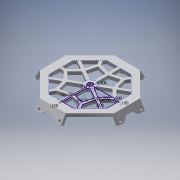
# Autodesk Inventor part: 4-Tool_Lower
Saved by Autodesk Inventor 2019 (Build 230136000, 136)
## iProperties
Created: 2021-01-31
Part Number: 4-Tool_Lower
Material: ABS Plastic
Document SubType Name: Modeling
Designer: zhanb
Density: 1.06 g/cm^3
Appearance: Smooth - White
Author: zhanb
Autodesk Inventor part; units mm, degrees
ref_plane "YZ Plane" through (0, 0, 0) normal (1, 0, 0) x (0, 1, 0)
ref_plane "XZ Plane" through (0, 0, 0) normal (0, 1, 0) x (-1, 0, 0)
ref_plane "XY Plane" through (0, 0, 0) normal (0, 0, 1) x (1, 0, 0)
sketch "Sketch1" plane through (0, 0, 0) normal (1, 0, 0) x (0, 1, 0)
  line L0 (76.2, -25.4) -> (50.8, -25.4) construction
  line L1 (50.8, -25.4) -> (50.8, 25.4) construction
  line L2 (50.8, 25.4) -> (76.2, 25.4) construction
  line L3 (76.2, 25.4) -> (76.2, -25.4) construction
  line L4 (76.2, -25.4) -> (50.8, 25.4) construction
  line L5 (50.8, -25.4) -> (76.2, 25.4) construction
  line L6 (76.2, 25.4) -> (-22.7867, 82.55) construction
  line L7 (-22.7867, 82.55) -> (-9.5885, 74.93)
  line L8 (-22.7867, 82.55) -> (-25.9617, 77.0507)
  line L9 (-25.9617, 77.0507) -> (-12.7635, 69.4307)
  line L10 (-9.5885, 74.93) -> (-12.7635, 69.4307) construction
  line L11 (-12.7635, 69.4307) -> (-12.7635, 57.15)
  line L12 (-12.7635, 57.15) -> (-6.4135, 57.15)
  line L13 (-6.4135, 57.15) -> (-6.4135, 73.0969)
  line L14 (-9.5885, 74.93) -> (-6.4135, 73.0969)
  point P0 (0, 0)
  point P1 (63.5, 0)
  point P2 (-16.1876, 78.74)
  dimension "d0" = 50.8
  dimension "d1" = 25.4
  dimension "d2" = 63.5
  dimension "d3" = 30
  dimension "d4" = 114.3
  dimension "d5" = 15.24
  dimension "d6" = 106.68
  dimension "d7" = 6.35
  dimension "d14" = 6.35
  dimension "d65" = 57.15
  constraints: 30 end point, 6 perpendicular, 3 midpoint, 2 parallel, 2 point on line, 1 collinear, 1 horizontal, 1 horizontal alignment, 1 vertical
  measures "d0" distance of L2.end L0.start
  measures "d1" distance of L1.end L2.end
  measures "d2" distance of point (0, 0) point (63.5, 0)
  measures "d3" angle of L2 L6
  measures "d4" distance of L2.end L6.end
  measures "d5" distance of L6.end L7.end
  measures "d6" distance of L2.end point (-16.188, 78.74)
  measures "d7" distance between parallel lines of L6 L9
  measures "d14" distance of L11.end L12.end
  measures "d65" distance from line of L12 point (0, 0)
extrude "Extrusion1" add sketch "Sketch1" along normal mid plane 50.8
pattern_circular "Circular Pattern1" count 4 over 360 about axis through (0, -10, 0) along (0, 1, 0) of "Extrusion1"
sketch "Sketch2" plane through (-25.4, -6.4135, 73.0969) normal (0, 1, 0) x (1, 0, 0)
  line L0 (50.8, 0) -> (0, 0) construction
  line L1 (50.8, 15.9469) -> (50.8, 0) construction
  line L2 (50.8, 15.9469) -> (0, 15.9469) construction
  line L3 (0, 0) -> (0, 15.9469) construction
  line L4 (-47.6969, 47.6969) -> (-47.6969, 98.4969) construction
  line L5 (-31.75, 47.6969) -> (-47.6969, 47.6969) construction
  line L6 (-31.75, 47.6969) -> (-31.75, 98.4969) construction
  line L7 (-47.6969, 98.4969) -> (-31.75, 98.4969) construction
  line L8 (-47.6969, 47.6969) -> (0, 0)
  line L9 (-44.0307, 47.6969) -> (-31.75, 47.6969) projected
  line L10 (-47.6969, 47.6969) -> (-31.75, 47.6969)
  line L11 (0, 0) -> (0, 15.9469)
  line L12 (0, 3.6662) -> (0, -3.9538) projected
  line L13 (0, 15.9469) -> (1.7277, 15.9469)
  line L14 (50.8, 15.9469) -> (0, 15.9469) projected
  line L15 (1.7277, 15.9469) -> (-31.75, 49.4246)
  line L16 (-31.75, 47.6969) -> (-31.75, 98.4969) projected
  line L17 (-31.75, 49.4246) -> (-31.75, 47.6969)
  point P0 (25.4, 73.0969)
  dimension "d64" = 57.15
  constraints: 12 end point, 2 collinear, 2 point on line, 1 horizontal, 1 parallel
  measures "d64" distance from line of L15 point (25.4, 73.097)
extrude "Extrusion2" add sketch "Sketch2" against normal up to surface (6.35 mm away)
sketch "Sketch3" plane through (-25.4, -22.7867, 82.55) normal (0, 0.5, 0.8660254) x (1, 0, 0)
  line L0 (50.8, 0) -> (0, 0) construction
  line L1 (10.16, 0) -> (18.034, 7.874)
  line L2 (18.034, 7.874) -> (32.766, 7.874)
  line L3 (32.766, 7.874) -> (40.64, 0)
  line L4 (10.16, 0) -> (40.64, 0)
  line L5 (5.08, 5.08) -> (45.72, 5.08) construction
  line L6 (0, 0) -> (0, 18.9062) construction
  line L7 (50.8, 18.9062) -> (50.8, 0) construction
  point P0 (25.4, 61.0089)
  point P1 (25.4, 7.874)
  point P2 (25.4, 0)
  dimension "d19" = 45
  dimension "d20" = 10.16
  dimension "d21" = 7.874
  dimension "d24" = 5.08
  dimension "d25" = 5.08
  dimension "d26" = 5.08
  constraints: 10 end point, 2 midpoint, 2 parallel, 2 point on line, 1 horizontal, 1 perpendicular, 1 vertical alignment
  measures "d19" angle of L0 L1
  measures "d20" distance of L0.end L1.start
  measures "d21" distance between parallel lines of L0 L2
  measures "d24" distance from line of L0 L5.start
  measures "d25" distance from line of L6 L5.start
  measures "d26" distance from line of L7 L5.end
extrude "Extrusion3" cut sketch "Sketch3" against normal through all
hole "Hole1" at (-20.32, -18.3873, 80.01) at (20.32, -18.3873, 80.01) direction (0, -0.5, -0.8660254) diameter 5.1562 end through all
sketch "Sketch5" plane through (0, 0, 0) normal (1, 0, 0) x (0, 1, 0)
  line L0 (-12.7635, 69.4307) -> (-25.9617, 77.0507) construction
  line L1 (-12.7635, 25.4) -> (-12.7635, 73.0969) projected
  line L2 (-19.1135, 73.0969) -> (-19.1135, 61.6669)
  line L3 (-19.1135, 61.6669) -> (-12.7635, 58.0007)
  line L4 (-12.7635, 69.4307) -> (-12.7635, 57.15) projected
  line L5 (-12.7635, 69.4307) -> (-19.1135, 73.0969)
  line L6 (-19.1426, 73.1137) -> (-25.9617, 77.0507) projected
  line L7 (-12.7635, 69.4307) -> (-12.7635, 58.0007)
  point P0 (0, 0)
  dimension "d34" = 6.35
  dimension "d35" = 11.43
  constraints: 8 end point, 2 collinear, 2 point on line, 1 parallel, 1 vertical
  measures "d34" distance between parallel lines of L1 L2
  measures "d35" distance of L2.start L2.end
extrude "Extrusion4" add sketch "Sketch5" along normal mid plane 5.08
pattern_circular "Circular Pattern2" count 4 over 360 about axis through (0, -10, 0) along (0, 1, 0) of "Extrusion4", "Extrusion3", "Hole1", "Extrusion2"
sketch "Sketch6" plane through (-25.4, -6.4135, 73.0969) normal (0, 1, 0) x (1, 0, 0)
  line L0 (20.6121, 70.3326) -> (20.6121, 75.8612) construction
  line L1 (20.6121, 75.8612) -> (25.4, 78.6255) construction
  line L2 (25.4, 78.6255) -> (30.1879, 75.8612) construction
  line L3 (30.1879, 75.8612) -> (30.1879, 70.3326) construction
  line L4 (30.1879, 70.3326) -> (25.4, 67.5683) construction
  line L5 (25.4, 67.5683) -> (20.6121, 70.3326) construction
  line L6 (82.55, 49.4246) -> (78.4987, 45.3733)
  line L7 (78.4987, 45.3733) -> (59.9942, 56.0569)
  line L8 (35.2679, 70.3326) -> (35.2679, 73.0969)
  line L9 (35.2679, 73.0969) -> (69.85, 73.0969)
  line L10 (82.55, 73.0969) -> (82.55, 70.5569) construction
  line L11 (32.7279, 65.9332) -> (52.8996, 54.2871)
  line L12 (74.7799, 41.6545) -> (56.8424, 23.717)
  line L13 (49.0723, 15.9469) -> (27.94, 15.9469)
  line L14 (27.94, 15.9469) -> (27.94, 34.6175)
  line L15 (27.94, 63.1689) -> (32.7279, 65.9332)
  line L16 (82.55, 96.7692) -> (82.55, 49.4246) construction
  line L17 (82.55, 49.4246) -> (53.1236, 19.9982) construction
  line L18 (49.0723, 15.9469) -> (1.7277, 15.9469) construction
  line L19 (1.7277, 15.9469) -> (-31.75, 49.4246) construction
  line L20 (-31.75, 49.4246) -> (-31.75, 96.7692) construction
  line L21 (-31.75, 96.7692) -> (1.7277, 130.2469) construction
  line L22 (1.7277, 130.2469) -> (49.0723, 130.2469) construction
  line L23 (49.0723, 130.2469) -> (82.55, 96.7692) construction
  line L24 (82.55, 96.7692) -> (82.55, 49.4246) construction
  line L25 (30.1879, 70.3326) -> (76.6393, 43.5139) construction
  line L26 (35.2679, 78.7941) -> (35.2679, 67.3997) construction
  line L27 (35.2679, 67.3997) -> (25.4, 61.7024) construction
  line L28 (25.4, 61.7024) -> (15.5321, 67.3997) construction
  line L29 (15.5321, 67.3997) -> (15.5321, 78.7941) construction
  line L30 (15.5321, 78.7941) -> (25.4, 84.4914) construction
  line L31 (25.4, 84.4914) -> (35.2679, 78.7941) construction
  line L32 (82.55, 70.5569) -> (74.4942, 70.5569)
  line L33 (74.4942, 70.5569) -> (59.9942, 56.0569)
  line L34 (55.4396, 58.6865) -> (69.85, 73.0969)
  line L35 (69.85, 73.0969) -> (82.55, 73.0969) construction
  line L36 (82.55, 70.5569) -> (82.55, 49.4246)
  line L37 (55.4396, 58.6865) -> (35.2679, 70.3326)
  line L38 (59.9942, 56.0569) -> (55.4396, 58.6865) construction
  line L39 (52.8996, 54.2871) -> (47.625, 34.6021)
  line L40 (47.625, 34.6021) -> (27.94, 39.8767)
  line L41 (57.4542, 51.6575) -> (52.1468, 31.8501)
  line L42 (52.1468, 31.8501) -> (56.8424, 23.717)
  line L43 (27.94, 34.6175) -> (47.7474, 29.3101)
  line L44 (47.7474, 29.3101) -> (53.1236, 19.9982)
  line L45 (54.983, 21.8576) -> (30.3339, 64.5511) construction
  line L46 (52.1468, 31.8501) -> (47.625, 34.6021) construction
  line L47 (47.625, 34.6021) -> (47.7474, 29.3101) construction
  line L48 (47.7474, 29.3101) -> (52.1468, 31.8501) construction
  line L49 (55.4396, 58.6865) -> (52.8996, 54.2871) construction
  line L50 (52.8996, 54.2871) -> (57.4542, 51.6575) construction
  line L51 (57.4542, 51.6575) -> (74.7799, 41.6545)
  line L52 (27.94, 39.8767) -> (27.94, 63.1689)
  line L53 (27.94, 34.6175) -> (27.94, 39.8767) construction
  line L54 (56.8424, 23.717) -> (53.1236, 19.9982) construction
  line L55 (53.1236, 19.9982) -> (49.0723, 15.9469) construction
  line L56 (53.1236, 19.9982) -> (49.0723, 15.9469)
  circle A0 centre (25.4, 73.0969) radius 4.7879
  line L57 (82.55, 49.4246) -> (49.0723, 15.9469) construction
  line L58 (27.94, 15.9469) -> (25.4, 15.9469)
  line L59 (25.4, 15.9469) -> (25.4, 61.7024)
  line L60 (25.4, 61.7024) -> (25.4, 68.309)
  line L61 (69.85, 73.0969) -> (82.55, 73.0969)
  line L62 (82.55, 73.0969) -> (82.55, 70.5569)
  line L63 (35.2679, 73.0969) -> (30.1879, 73.0969)
  arc A1 (25.4, 68.309) -> (30.1879, 73.0969) centre (25.4, 73.0969) ccw
  line L64 (53.1236, 19.9982) -> (56.8424, 23.717)
  line L65 (78.4987, 45.3733) -> (74.7799, 41.6545)
  point P0 (25.4, 73.0969)
  point P1 (27.794, 68.9505)
  point P2 (27.7939, 77.2434)
  dimension "d41" = 9.5758
  dimension "d42" = 2.54
  dimension "d43" = 5.08
  dimension "d45" = 30
  dimension "d46" = 5.08
  dimension "d48" = 5.08
  dimension "d49" = 2.54
  dimension "d50" = 5.08
  dimension "d51" = 5.08
  dimension "d52" = 5.08
  dimension "d61" = 12.7
  constraints: 128 end point, 17 parallel, 13 collinear, 13 point on line, 7 midpoint, 7 perpendicular, 5 coincident, 5 point on circle, 5 vertical, 3 horizontal, 2 centre point, 1 equal length, 46 other
  measures "d41" distance between parallel lines of L0 L3
  measures "d42" distance from line of L4.end L14
  measures "d43" distance between parallel lines of L7 L11
  measures "d45" angle of L9 L25
  measures "d46" distance between parallel lines of L26 L3
  measures "d48" distance between parallel lines of L34 L33
  measures "d49" distance between parallel lines of L35 L32
  measures "d50" distance between parallel lines of L44 L42
  measures "d51" distance between parallel lines of L39 L41
  measures "d52" distance between parallel lines of L43 L40
  measures "d61" distance of L10.start L9.end
extrude "Extrusion6" add sketch "Sketch6" against normal up to surface (6.35 mm away) contours L65 L51 L41 L42 L64 L44 L43 L14 L58 L59 L60 A0 L63 L8 L37 L34 L61 L62 L32 L33 L7
mirror "Mirror1" about plane through (0, 0, 0) normal (1, 0, 0) of "Extrusion6"
mirror "Mirror2" about plane through (0, 0, 0) normal (0, 0, 1) of "Extrusion6", "Mirror1"
fillet "Fillet2" radius 1.5875 50 edges at (-2.54, -9.5885, -33.2202) (-22.225, -9.5885, -38.4948) (-2.54, -9.5885, -9.928) (-2.54, -9.5885, -38.4795) (-22.3474, -9.5885, -43.7868) (-26.7468, -9.5885, -41.2468) (-32.0542, -9.5885, -21.4394) (-7.3279, -9.5885, -7.1637) (-27.4996, -9.5885, -18.8098) (-34.5942, -9.5885, -17.04) (-49.0942, -9.5885, -2.54) (-30.0396, -9.5885, -14.4104) (22.225, -9.5885, -38.4948) (2.54, -9.5885, -33.2202) (2.54, -9.5885, -9.928) (2.54, -9.5885, -38.4795) (22.3474, -9.5885, -43.7868) (26.7468, -9.5885, -41.2468) (32.0542, -9.5885, -21.4394) (7.3279, -9.5885, -7.1637) (27.4996, -9.5885, -18.8098) (34.5942, -9.5885, -17.04) (49.0942, -9.5885, -2.54) (30.0396, -9.5885, -14.4104) (2.54, -9.5885, 33.2202) (22.225, -9.5885, 38.4948) (2.54, -9.5885, 9.928) (2.54, -9.5885, 38.4795) (22.3474, -9.5885, 43.7868) (26.7468, -9.5885, 41.2468) (32.0542, -9.5885, 21.4394) (7.3279, -9.5885, 7.1637) (27.4996, -9.5885, 18.8098) (34.5942, -9.5885, 17.04) (49.0942, -9.5885, 2.54) (30.0396, -9.5885, 14.4104) (9.8679, -9.5885, 2.7643) (-22.225, -9.5885, 38.4948) (-2.54, -9.5885, 33.2202) (-2.54, -9.5885, 9.928) (-2.54, -9.5885, 38.4795) (-22.3474, -9.5885, 43.7868) (-26.7468, -9.5885, 41.2468) (-32.0542, -9.5885, 21.4394) (-7.3279, -9.5885, 7.1637) (-27.4996, -9.5885, 18.8098) (-34.5942, -9.5885, 17.04) (-49.0942, -9.5885, 2.54) (-30.0396, -9.5885, 14.4104) (-9.8679, -9.5885, 2.7643)
fillet "Fillet2" radius 1.5875 32 edges at (23.6723, -9.5885, 57.15) (27.7236, -9.5885, 53.0987) (2.54, -9.5885, 57.15) (-2.54, -9.5885, 57.15) (-23.6723, -9.5885, 57.15) (-27.7236, -9.5885, 53.0987) (-31.4424, -9.5885, 49.3799) (-49.3799, -9.5885, 31.4424) (-53.0987, -9.5885, 27.7236) (-57.15, -9.5885, 23.6723) (-57.15, -9.5885, 2.54) (-57.15, -9.5885, -2.54) (-57.15, -9.5885, -23.6723) (-53.0987, -9.5885, -27.7236) (-49.3799, -9.5885, -31.4424) (-31.4424, -9.5885, -49.3799) (-27.7236, -9.5885, -53.0987) (-2.54, -9.5885, -57.15) (2.54, -9.5885, -57.15) (23.6723, -9.5885, -57.15) (27.7236, -9.5885, -53.0987) (49.3799, -9.5885, -31.4424) (57.15, -9.5885, -23.6723) (57.15, -9.5885, -2.54) (57.15, -9.5885, 2.54) (57.15, -9.5885, 23.6723) (53.0987, -9.5885, 27.7236) (49.3799, -9.5885, 31.4424) (31.4424, -9.5885, 49.3799) (-23.6723, -9.5885, -57.15) (31.4424, -9.5885, -49.3799) (53.0987, -9.5885, -27.7236)
fillet "Fillet3" radius 1.5875 8 edges at (13.97, -12.7635, 69.4307) (-13.97, -12.7635, 69.4307) (69.4307, -12.7635, 13.97) (69.4307, -12.7635, -13.97) (13.97, -12.7635, -69.4307) (-13.97, -12.7635, -69.4307) (-69.4307, -12.7635, 13.97) (-69.4307, -12.7635, -13.97)
equation "\"d5\" = -2 * d6 + 2 * d4"
equation "\"d26\" = d25"
equation "\"d48\" = d43"
equation "\"d51\" = d50"
equation "\"d52\" = d50"
body "Solid1"
